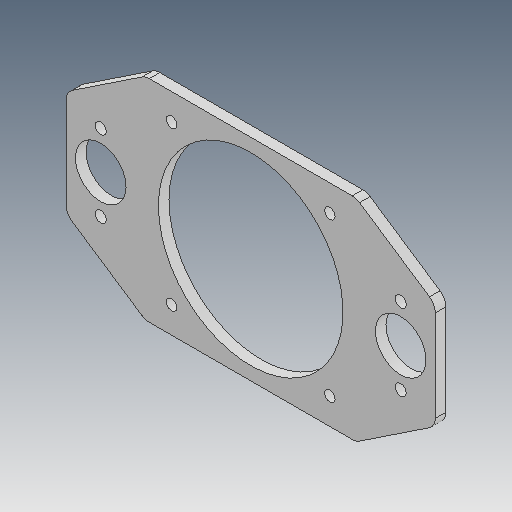
# Autodesk Inventor part: suporte-superior
Saved by Autodesk Inventor 2020 (Build 240168000, 168)
## iProperties
Created: 2022-07-20
Part Number: suporte-superior
Material: Genérico
Document SubType Name: Modeling
Designer: gabri
Density: 1 g/cm^3
Appearance: Padrão
Author: gabri
Autodesk Inventor part; units mm, degrees
ref_plane "YZ Plane" through (0, 0, 0) normal (1, 0, 0) x (0, 1, 0)
ref_plane "XZ Plane" through (0, 0, 0) normal (0, 1, 0) x (-1, 0, 0)
ref_plane "XY Plane" through (0, 0, 0) normal (0, 0, 1) x (1, 0, 0)
ref_plane "Plano de trabalho1" through (0, 0, 0) normal (0, 0, 1) x (1, 0, 0)
sketch "Esboço1" plane through (0, 0, 0) normal (0, 0, 1) x (1, 0, 0)
  arc A0 (-40, -30) -> (-30, -40) centre (-30, -30) ccw projected
  line L0 (30, -40) -> (-30, -40) projected
  line L1 (40, 30) -> (40, -30) projected
  arc A1 (40, 30) -> (30, 40) centre (30, 30) ccw projected
  line L2 (-30, 40) -> (30, 40) projected
  arc A2 (-30, 40) -> (-40, 30) centre (-30, 30) ccw projected
  line L3 (-40, -30) -> (-40, 30) projected
  circle A3 centre (0, 0) radius 5 projected
  circle A4 centre (0, 0) radius 35
  circle A5 centre (30, 30) radius 2
  circle A6 centre (30, -30) radius 2
  circle A7 centre (-30, -30) radius 2
  circle A8 centre (-30, 30) radius 2
  line L4 (0, 0) -> (88.4205, 0)
  circle A9 centre (56.873, 0) radius 9.6
  circle A10 centre (56.873, 0) radius 24.3683
  line L5 (70, -20) -> (70, 13.4311)
  line L6 (0, -54.5393) -> (0, 0)
  line L7 (0, 0) -> (97.6155, 0)
  line L8 (40, -30) -> (40, -40)
  line L9 (40, -40) -> (30, -40)
  line L10 (40, -40) -> (70, -20)
  circle A11 centre (56.873, -14.5) radius 2.1
  point P0 (0, 0)
  point P1 (70, 0)
  point P2 (66.473, 0)
  point P3 (47.273, 0)
  point P4 (5, 0)
  point P5 (0, -5)
  point P6 (0, -40)
  point P7 (35, 0)
  point P8 (0, -35)
  dimension "d0" = 70
  dimension "d3" = 4
  dimension "d4" = 4
  dimension "d5" = 4
  dimension "d6" = 4
  dimension "d7" = 19.2
  dimension "d8" = 30
  dimension "d9" = 20
  dimension "d12" = 4.2
  dimension "d13" = 14.5
  dimension "d14" = 16.873
  dimension "d15" = 16.873
  constraints: 14 end point, 8 centre point, 5 coincident, 2 point on line, 2 vertical, 1 collinear, 1 horizontal, 1 perpendicular
  measures "d0" diameter of A4
  measures "d3" diameter of A5
  measures "d4" diameter of A6
  measures "d5" diameter of A7
  measures "d6" diameter of A8
  measures "d7" diameter of A9
  measures "d8" distance between parallel lines of L1 L5
  measures "d9" distance from line of L4 L5.start
  measures "d12" diameter of A11
  measures "d13" distance of A9.centre A11.centre
  measures "d14" distance from line of L1 A9.centre
  measures "d15" distance from line of L1 A11.centre
extrude "Extrusão2" add sketch "Esboço1" along normal blind 4 contours L6 A4 A10 L1 L8 L9 L0 | L8 L1 A10 L10 | A4 L4 L1 A10 | A10 L1 L4 A9 L5 L10 picked at (39.1782, -10.8029)
mirror "Espelhamento1" about plane through (70, 0, 0) normal (0, 1, 0) of "Extrusão2"
mirror "Espelhamento2" about plane through (0, 35, 0) normal (-1, 0, 0) of "Extrusão2", "Espelhamento1"
fillet "Arredondamento1" radius 5 8 edges at (40, -40, 2) (70, -20, 2) (70, 20, 2) (40, 40, 2) (-40, 40, 2) (-70, 20, 2) (-70, -20, 2) (-40, -40, 2)
equation "\"d3\" = d6"
equation "\"d4\" = d6"
equation "\"d5\" = d6"
equation "\"d15\" = d14"
